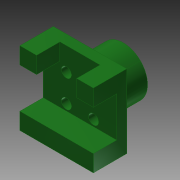
# Autodesk Inventor part: coupler1
Saved by Autodesk Inventor 2013 (Build 170138000, 138)
## iProperties
Created: 2014-10-09
Part Number: coupler1
Material: Generic
Document SubType Name: Modeling
Designer: Masta
Density: 1 g/cm^3
Author: Masta
Autodesk Inventor part; units mm, degrees
ref_plane "YZ Plane" through (0, 0, 0) normal (1, 0, 0) x (0, 1, 0)
ref_plane "XZ Plane" through (0, 0, 0) normal (0, 1, 0) x (-1, 0, 0)
ref_plane "XY Plane" through (0, 0, 0) normal (0, 0, 1) x (1, 0, 0)
sketch "Sketch1" plane through (0, 0, 0) normal (0, 1, 0) x (-1, 0, 0)
  circle A0 centre (0, 0) radius 7.25
  line L0 (0, 0) -> (7.25, 0) construction
  line L1 (0, 0) -> (0, 7.25) construction
  line L2 (11, -11) -> (-11, -11)
  line L3 (-11, -11) -> (-11, 11)
  line L4 (-11, 11) -> (11, 11)
  line L5 (11, 11) -> (11, -11)
  line L6 (11, -11) -> (-11, 11) construction
  line L7 (-11, -11) -> (11, 11) construction
  line L8 (-11, 11) -> (-6, 11)
  line L9 (-6, 11) -> (-6, 6)
  line L10 (-6, 6) -> (-11, 6)
  line L11 (-11, 6) -> (-11, 11)
  line L12 (11, 11) -> (6, 11)
  line L13 (6, 11) -> (6, 6)
  line L14 (6, 6) -> (11, 6)
  line L15 (11, 6) -> (11, 11)
  line L16 (-11, -11) -> (11, -11)
  line L17 (11, -11) -> (11, -6)
  line L18 (11, -6) -> (-11, -6)
  line L19 (-11, -6) -> (-11, -11)
  line L20 (-6, 6) -> (6, 6) construction
  line L21 (4.0659, -4.0659) -> (-4.0659, -4.0659) construction
  line L22 (-4.0659, -4.0659) -> (-4.0659, 4.0659) construction
  line L23 (-4.0659, 4.0659) -> (4.0659, 4.0659) construction
  line L24 (4.0659, 4.0659) -> (4.0659, -4.0659) construction
  line L25 (4.0659, -4.0659) -> (-4.0659, 4.0659) construction
  line L26 (-4.0659, -4.0659) -> (4.0659, 4.0659) construction
  line L27 (-5.1265, 5.1265) -> (-4.0659, 4.0659) construction
  circle A1 centre (-4.0659, 4.0659) radius 1.5
  circle A2 centre (4.0659, 4.0659) radius 1.5
  circle A3 centre (4.0659, -4.0659) radius 1.5
  circle A4 centre (-4.0659, -4.0659) radius 1.5
  dimension "d0" = 14.5
  dimension "d3" = 12
  dimension "d4" = 5
  dimension "d9" = 1.5
  constraints: 56 end point, 10 parallel, 8 perpendicular, 6 horizontal, 5 coincident, 5 point on line, 4 centre point, 4 midpoint, 3 point on circle, 3 tangent, 1 collinear, 4 other
  measures "d0" diameter of A0
  measures "d3" distance between parallel lines of L10 L18
  measures "d4" distance of L18.end L2.end
  measures "d9" distance of L27.start L22.end
extrude "Extrusion1" add sketch "Sketch1" along normal blind 10 contours A0 L18 | A0 L18
extrude "Extrusion2" add sketch "Sketch1" against normal blind 3 contours A0 L18 | A0 L18 L3 L10 L9 L4 L13 L14 L5 picked at (1.037, 0.9609)
extrude "Extrusion3" add sketch "Sketch1" against normal blind 10 contours L18 L5 L2 L3 A0 | A0 L18 | L14 L13 L4 L5 | L3 L4 L9 L10 picked at (0.8459, -6.2638)
body "Solid1"
